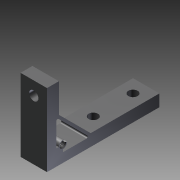
# Autodesk Inventor part: HBLTF6-C_
Saved by Autodesk Inventor 2011 SP1 (Build 150282100, 282)
## iProperties
Created: 2016-11-23
Part Number: HBLTF6-C_
Catalog Web Link: www.cadenas.de
Description: HBLTS6, HBLTSB6, HBLTD6-50, HBLFTD6-50, HBLFTDM6-50,HBLFTDB6-50, HBLTD6, HBLTDB6, HBLFTD6-50, HBLFTDM6, HBLFTDB6, HBLTT6, HBLTSW6, HBLTDW6, HBLTTW6, HBLTFW6hblts6-Thick Brackets for Slot Width 8 Frames - For 30, 50, 60mm Sections
Vendor: MISUMI
Document SubType Name: Modeling
Designer: psAdmin
Manufacturer: MISUMI
Mass: 22.6313 g
Surface Area: 100.055 cm^2
Volume: 22.6313 cm^3
Density: 1 g/cm^3
Category: PARTsolutions
Company: MISUMI
Title: HBLTF6-C_
Author: Cadenas PARTsolutions
Comments: Thick Brackets for Slot Width 8 Frames - For 30, 50, 60mm Sections
PSOL_IDENT_0: {$CADENAS_DATA\23d-libs\misumi\metric\38_al_extrusions_blackets\6\hblts6.prj},321 {VTYP=3D},{NB=HBLT
PSOL_IDENT_1: F6-C_},{LINA=HBLTF6-C_},{NN=HBLTS6, HBLTSB6, HBLTD6-50, HBLFTD6-50, HBLFTDM6-50,HBLFTDB6-50, HBLTD6,
PSOL_IDENT_2: HBLTDB6, HBLFTD6-50, HBLFTDM6, HBLFTDB6, HBLTT6, HBLTSW6, HBLTDW6, HBLTTW6, HBLTFW6hblts6},{DATE=17
PSOL_IDENT_3: .06.2016 05:53:16},{GEOMDATE=18.02.2013 03:40:00},{VERSION=},{LINEID=240},{LINESUBID=-1},{WBVAR=ALT1
PSOL_IDENT_4: }  {NB=HBLTF6-C_},{LINA=HBLTF6-C_},{KT=7},{PN=HBLTF6-C},{TP=HBLTF6},{HDISY=30},{HDISZ=30},{NOH=1},{N
PSOL_IDENT_5: OHV=2},{ST=Alumite},{TYPE=HBLTF6},{FEAT=Thick Bracket},{ALT1=-C},{NON=4},{AL=1764},{W=20},{L=55},{T=
PSOL_IDENT_6: 9},{HPOS=0},{L1=45},{H=85},{H1=45},{H2=33},{DIA=7},{R=3.1},{R1=1},{ANGLE=45},{VER=1},{PR=7},{T1=2.0}
PSOL_IDENT_7: ,{T2=7},{DPOS=12}
NN: HBLTS6, HBLTSB6, HBLTD6-50, HBLFTD6-50, HBLFTDM6-50,HBLFTDB6-50, HBLTD6, HBLTDB6, HBLFTD6-50, HBLFTDM6, HBLFTDB6, HBLTT6, HBLTSW6, HBLTDW6, HBLTTW6, HBLTFW6hblts6
NT: Thick Brackets for Slot Width 8 Frames - For 30, 50, 60mm Sections
NB: HBLTF6-C_
NBSYN: $PN._
LINA: HBLTF6-C_
PN: HBLTF6-C
TP: HBLTF6
HDISY: 30
ST: Clear Anodizing
FEAT: Thick Bracket
ALT1: with C (Mounting Holes for Cover)
NON: 4
AL: 1764
SUPPLIER: MISUMI
ARTICLENO: HBLTF6-C_
BOMINFO: HBLTF6-C_
CREATOR: CADENAS GmbH
Autodesk Inventor part; units mm, degrees
sketch "Sketch_1" plane through (0, 0, 0) normal (1, 0, 0) x (0, 1, 0)
  line L0 (0, 55) -> (0, 0)
  line L1 (0, 0) -> (85, 0)
  line L2 (85, 0) -> (85, 9)
  line L3 (85, 9) -> (33, 9)
  line L4 (33, 9) -> (9, 33)
  line L5 (9, 33) -> (9, 55)
  line L6 (9, 55) -> (0, 55)
  arc A0 (8.7071, 30.4645) -> (7, 29.7574) centre (8, 29.7574) ccw
  line L7 (7, 29.7574) -> (7, 12)
  line L8 (7, 12) -> (8.9, 12)
  arc A1 (12.5383, 15.0529) -> (8.9, 12) centre (12, 12) ccw
  line L9 (12.5383, 15.0529) -> (12.3647, 14.0681)
  arc A2 (12.3647, 14.0681) -> (14.0681, 12.3647) centre (12.5843, 12.5843) ccw
  line L10 (14.0681, 12.3647) -> (15.0529, 12.5383)
  arc A3 (12, 8.9) -> (15.0529, 12.5383) centre (12, 12) ccw
  line L11 (12, 8.9) -> (12, 7)
  line L12 (12, 7) -> (29.7574, 7)
  arc A4 (29.7574, 7) -> (30.4645, 8.7071) centre (29.7574, 8) ccw
  line L13 (30.4645, 8.7071) -> (8.7071, 30.4645)
  constraints: 28 end point, 10 point on circle, 5 centre point
extrude "Extrusion1" add sketch "Sketch_1" along normal mid plane 20
sketch "Sketch_10" plane through (0, 12, 0) normal (0, 1, 0) x (1, 0, 0)
  line L0 (-10, -12) -> (10, -12)
  line L1 (10, -12) -> (10, -14.5)
  line L2 (10, -14.5) -> (9.567, -14.067)
  line L3 (9.567, -14.067) -> (-9.567, -14.067)
  line L4 (-9.567, -14.067) -> (-10, -14.5)
  line L5 (-10, -14.5) -> (-10, -12)
  line L6 (-10, -12) -> (10, -12)
  constraints: 14 end point
revolve "Revolution1" cut sketch "Sketch_10" angle 360 about axis through (-10, 12, 12) along (-1, 0, 0)
thread "Thread1" size "M5x0.8" class "6H" standard "ISO Metric profile" full length
sketch "Sketch3" plane through (10, 0, 0) normal (0, 0, -1) x (-1, 0, 0)
  point P0 (10, 45)
hole "Hole1" at (0, 45, 0) direction (0, 0, 1) diameter 7 depth 9
sketch "Sketch4" plane through (-10, 0, 55) normal (0, -1, 0) x (1, 0, 0)
  point P0 (10, -10)
hole "Hole2" at (0, 0, 45) direction (0, 1, 0) diameter 7 depth 9
sketch "Sketch5" plane through (10, 0, 0) normal (0, 0, -1) x (-1, 0, 0)
  point P0 (10, 75)
hole "Hole3" at (0, 75, 0) direction (0, 0, 1) diameter 7 depth 9
ref_plane "a10_to_bolt_XY" through (0, 9, 75) normal (0, 1, 0) x (1, 0, 0)
ref_plane "a10_to_bolt_YZ" through (0, 9, 75) normal (1, 0, 0) x (0, 0, -1)
ref_plane "a10_to_bolt_ZX" through (0, 9, 75) normal (0, 0, -1) x (0, 1, 0)
ref_plane "a11_to_bolt_XY" through (0, 75, 9) normal (0, 0, 1) x (1, 0, 0)
ref_plane "a11_to_bolt_YZ" through (0, 75, 9) normal (1, 0, 0) x (0, 1, 0)
ref_plane "a11_to_bolt_ZX" through (0, 75, 9) normal (0, 1, 0) x (0, 0, 1)
ref_plane "a13_to_bolt_XY" through (20, 75, 9) normal (0, 0, 1) x (1, 0, 0)
ref_plane "a13_to_bolt_YZ" through (20, 75, 9) normal (1, 0, 0) x (0, 1, 0)
ref_plane "a13_to_bolt_ZX" through (20, 75, 9) normal (0, 1, 0) x (0, 0, 1)
ref_plane "a14_to_bolt_XY" through (-20, 75, 9) normal (0, 0, 1) x (1, 0, 0)
ref_plane "a14_to_bolt_YZ" through (-20, 75, 9) normal (1, 0, 0) x (0, 1, 0)
ref_plane "a14_to_bolt_ZX" through (-20, 75, 9) normal (0, 1, 0) x (0, 0, 1)
ref_plane "a15_to_bolt_XY" through (20, 45, 9) normal (0, 0, 1) x (1, 0, 0)
ref_plane "a15_to_bolt_YZ" through (20, 45, 9) normal (1, 0, 0) x (0, 1, 0)
ref_plane "a15_to_bolt_ZX" through (20, 45, 9) normal (0, 1, 0) x (0, 0, 1)
ref_plane "a16_to_bolt_XY" through (-20, 45, 9) normal (0, 0, 1) x (1, 0, 0)
ref_plane "a16_to_bolt_YZ" through (-20, 45, 9) normal (1, 0, 0) x (0, 1, 0)
ref_plane "a16_to_bolt_ZX" through (-20, 45, 9) normal (0, 1, 0) x (0, 0, 1)
ref_plane "a17_to_bolt_XY" through (20, 9, 75) normal (0, 1, 0) x (1, 0, 0)
ref_plane "a17_to_bolt_YZ" through (20, 9, 75) normal (1, 0, 0) x (0, 0, -1)
ref_plane "a17_to_bolt_ZX" through (20, 9, 75) normal (0, 0, -1) x (0, 1, 0)
ref_plane "a18_XY" through (-20, 9, 75) normal (0, 1, 0) x (1, 0, 0)
ref_plane "a18_YZ" through (-20, 9, 75) normal (1, 0, 0) x (0, 0, -1)
ref_plane "a18_ZX" through (-20, 9, 75) normal (0, 0, -1) x (0, 1, 0)
ref_plane "a19_to_bolt_XY" through (20, 9, 45) normal (0, 1, 0) x (1, 0, 0)
ref_plane "a19_to_bolt_YZ" through (20, 9, 45) normal (1, 0, 0) x (0, 0, -1)
ref_plane "a19_to_bolt_ZX" through (20, 9, 45) normal (0, 0, -1) x (0, 1, 0)
ref_plane "a1_to_bolt_XY" through (0, 45, 9) normal (0, 0, 1) x (1, 0, 0)
ref_plane "a1_to_bolt_YZ" through (0, 45, 9) normal (1, 0, 0) x (0, 1, 0)
ref_plane "a1_to_bolt_ZX" through (0, 45, 9) normal (0, 1, 0) x (0, 0, 1)
ref_plane "a20_to_bolt_XY" through (-20, 9, 45) normal (0, 1, 0) x (1, 0, 0)
ref_plane "a20_to_bolt_YZ" through (-20, 9, 45) normal (1, 0, 0) x (0, 0, -1)
ref_plane "a20_to_bolt_ZX" through (-20, 9, 45) normal (0, 0, -1) x (0, 1, 0)
ref_plane "a2_to_bolt_XY" through (0, 9, 45) normal (0, 1, 0) x (1, 0, 0)
ref_plane "a2_to_bolt_YZ" through (0, 9, 45) normal (1, 0, 0) x (0, 0, -1)
ref_plane "a2_to_bolt_ZX" through (0, 9, 45) normal (0, 0, -1) x (0, 1, 0)
ref_plane "a3_to_bolt_XY" through (0, 75, 9) normal (0, 0, 1) x (1, 0, 0)
ref_plane "a3_to_bolt_YZ" through (0, 75, 9) normal (1, 0, 0) x (0, 1, 0)
ref_plane "a3_to_bolt_ZX" through (0, 75, 9) normal (0, 1, 0) x (0, 0, 1)
ref_plane "a4_to_bolt_XY" through (0, 75, 9) normal (0, 0, 1) x (1, 0, 0)
ref_plane "a4_to_bolt_YZ" through (0, 75, 9) normal (1, 0, 0) x (0, 1, 0)
ref_plane "a4_to_bolt_ZX" through (0, 75, 9) normal (0, 1, 0) x (0, 0, 1)
ref_plane "a5_to_bolt_XY" through (0, 9, 75) normal (0, 1, 0) x (1, 0, 0)
ref_plane "a5_to_bolt_YZ" through (0, 9, 75) normal (1, 0, 0) x (0, 0, -1)
ref_plane "a5_to_bolt_ZX" through (0, 9, 75) normal (0, 0, -1) x (0, 1, 0)
ref_plane "a6_to_bolt_XY" through (0, 9, 75) normal (0, 1, 0) x (1, 0, 0)
ref_plane "a6_to_bolt_YZ" through (0, 9, 75) normal (1, 0, 0) x (0, 0, -1)
ref_plane "a6_to_bolt_ZX" through (0, 9, 75) normal (0, 0, -1) x (0, 1, 0)
ref_plane "a7_to_bolt_XY" through (0, 75, 9) normal (0, 0, 1) x (1, 0, 0)
ref_plane "a7_to_bolt_YZ" through (0, 75, 9) normal (1, 0, 0) x (0, 1, 0)
ref_plane "a7_to_bolt_ZX" through (0, 75, 9) normal (0, 1, 0) x (0, 0, 1)
ref_plane "a8_to_bolt_XY" through (0, 75, 9) normal (0, 0, 1) x (1, 0, 0)
ref_plane "a8_to_bolt_YZ" through (0, 75, 9) normal (1, 0, 0) x (0, 1, 0)
ref_plane "a8_to_bolt_ZX" through (0, 75, 9) normal (0, 1, 0) x (0, 0, 1)
ref_plane "a9_to_bolt_XY" through (0, 9, 75) normal (0, 1, 0) x (1, 0, 0)
ref_plane "a9_to_bolt_YZ" through (0, 9, 75) normal (1, 0, 0) x (0, 0, -1)
ref_plane "a9_to_bolt_ZX" through (0, 9, 75) normal (0, 0, -1) x (0, 1, 0)
ref_plane "bracket_to_dummy_XY" through (0, 0, 0) normal (0, 1, 0) x (1, 0, 0)
ref_plane "bracket_to_dummy_YZ" through (0, 0, 0) normal (1, 0, 0) x (0, 0, -1)
ref_plane "bracket_to_dummy_ZX" through (0, 0, 0) normal (0, 0, -1) x (0, 1, 0)
ref_plane "h12_to_bolt_XY" through (0, 9, 75) normal (0, 1, 0) x (1, 0, 0)
ref_plane "h12_to_bolt_YZ" through (0, 9, 75) normal (1, 0, 0) x (0, 0, -1)
ref_plane "h12_to_bolt_ZX" through (0, 9, 75) normal (0, 0, -1) x (0, 1, 0)
body "Solid1"
